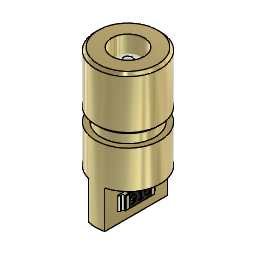
5mW (Autodesk Fusion 360 design; units mm, degrees)
Autodesk Fusion 360 part; units mm, degrees
note: some values were not read from the file. Set by a fixed rule: which sketch regions a step uses.
sketch "Sketch1" plane through (0, 0, 0) normal (0, 0, 1) x (1, 0, 0)
  circle A0 centre (0, 0) radius 3
  dimension "d1" = 6
  constraint coincident A0.centre origin
  measures "d1" diameter of A0
extrude "Extrude1" add sketch "Sketch1" along normal blind 7 makes body 1
sketch "Sketch2" plane through (0, 0, 7) normal (0, 0, 1) x (-1, 0, 0)
  circle A0 centre (0, 0) radius 3
  circle A1 centre (0, 0) radius 2.5
  dimension "d4" = 5
  constraint concentric A0 A1
  measures "d4" diameter of A1
extrude "Extrude2" add sketch "Sketch2" along normal blind 1 contours A1 bodies 1
sketch "Sketch3" plane through (0, 0, 8) normal (0, 0, 1) x (-1, 0, 0)
  circle A0 centre (0, 0) radius 2.5
  circle A1 centre (0, 0) radius 3
  dimension "d7" = 6
  constraint concentric A0 A1
  measures "d7" diameter of A1
extrude "Extrude3" add sketch "Sketch3" along normal blind 5 contours A0 | A1 bodies 1
sketch "Sketch4" plane through (0, 0, 0) normal (0, 0, -1) x (1, 0, 0)
  circle A0 centre (0, 0) radius 3
  line L0 (-0.75, 2.9047) -> (-0.75, -2.9047)
  line L1 (0.75, 2.9047) -> (0.75, -2.9047)
  dimension "d10" = 0.75
  dimension "d11" = 0.75
  constraint coincident A0 L0.start
  constraint coincident A0 L0.end
  constraint vertical L0
  constraint coincident A0 L1.start
  constraint coincident A0 L1.end
  constraint parallel L0 L1
  measures "d10" distance of A0.centre L0
  measures "d11" distance of A0.centre L1
extrude "Extrude4" cut sketch "Sketch4" against normal blind 3.5 contours A0 L1 | A0 L0 bodies 1
sketch "Sketch5" plane through (0, 0, 13) normal (0, 0, 1) x (-1, 0, 0)
  circle A0 centre (0, 0) radius 3
  circle A1 centre (0, 0) radius 1.5
  dimension "d14" = 3
  constraint coincident A0.centre A1.centre
  measures "d14" diameter of A1
extrude "Extrude5" cut sketch "Sketch5" against normal blind 3 contours A1 bodies 1
sketch "Sketch6" plane through (0, 0, 10) normal (0, 0, 1) x (-1, 0, 0)
  circle A0 centre (0, 0) radius 1.5
  circle A1 centre (0, 0) radius 1.4
  dimension "d17" = 2.8
  constraint concentric A0 A1
  measures "d17" diameter of A1
extrude "Extrude6" add sketch "Sketch6" along normal blind 2 separate body contours A1 makes body 2
fillet "Fillet1" radius 1 1 edges at (1.3053, 0.5063, 12) on bodies 2
chamfer "Chamfer1" distance 0.25 angle 45 2 edges at (2.797, 1.0848, 13) (2.797, 1.0848, 8) on bodies 1
sketch "Sketch7" plane through (-0.75, 0, 0) normal (-1, 0, 0) x (0, -1, 0)
  line L0 (-2.9047, 0) -> (2.9047, 0)
  line L1 (2.9047, 0) -> (2.9047, 3.5)
  line L2 (2.9047, 3.5) -> (-2.9047, 3.5)
  line L3 (-2.9047, 3.5) -> (-2.9047, 0)
  circle A0 centre (0, 1.6) radius 1
  dimension "d23" = 2
  dimension "d48" = 2.9047
  dimension "d49" = 1.6
  measures "d23" diameter of A0
  measures "d48" distance of L1 A0.centre
  measures "d49" distance of L0 A0.centre
extrude "Extrude7" add sketch "Sketch7" along normal blind 0.5 contours A0 bodies 1
fillet "Fillet2" radius 0.75 1 edges at (-1.25, 0.9323, 1.2384) on bodies 1
sketch "Sketch8" plane through (0.75, 0, 0) normal (1, 0, 0) x (0, 1, 0)
  line L0 (-2.9047, 0) -> (2.9047, 0)
  line L1 (2.9047, 0) -> (2.9047, 3.5)
  line L2 (2.9047, 3.5) -> (-2.9047, 3.5)
  line L3 (-2.9047, 3.5) -> (-2.9047, 0)
  line L4 (1.75, 1.0641) -> (-1.75, 1.0641)
  line L5 (-1.75, 1.0641) -> (-1.75, 2.3141)
  line L6 (-1.75, 2.3141) -> (1.75, 2.3141)
  line L7 (1.75, 2.3141) -> (1.75, 1.0641)
  line L8 (1.75, 1.0641) -> (-1.75, 2.3141) construction
  line L9 (-1.75, 1.0641) -> (1.75, 2.3141) construction
  line L10 (-1.75, 2.3141) -> (-1.375, 2.3141)
  line L11 (-1.375, 2.3141) -> (-1.375, 1.0641)
  line L12 (-1.375, 1.0641) -> (-1.75, 1.0641)
  line L13 (-1.75, 1.0641) -> (-1.75, 2.3141)
  line L14 (1.75, 2.3141) -> (1.375, 2.3141)
  line L15 (1.375, 2.3141) -> (1.375, 1.0641)
  line L16 (1.375, 1.0641) -> (1.75, 1.0641)
  line L17 (1.75, 1.0641) -> (1.75, 2.3141)
  line L18 (-1.375, 2.3141) -> (-1, 2.3141)
  line L19 (-1, 2.3141) -> (-1, 1.0641)
  line L20 (-1, 1.0641) -> (-1.375, 1.0641)
  line L21 (-1.375, 1.0641) -> (-1.375, 2.3141)
  line L22 (1.375, 2.3141) -> (1, 2.3141)
  line L23 (1, 2.3141) -> (1, 1.0641)
  line L24 (1, 1.0641) -> (1.375, 1.0641)
  line L25 (1.375, 1.0641) -> (1.375, 2.3141)
  line L26 (-1, 2.3141) -> (1, 2.3141)
  line L27 (1, 2.3141) -> (1, 2.3151)
  line L28 (1, 2.3151) -> (-1, 2.3151)
  line L29 (-1, 2.3151) -> (-1, 2.3141)
  line L30 (1, 1.0641) -> (-1, 1.0641)
  line L31 (-1, 1.0641) -> (-1, 1.0631)
  line L32 (-1, 1.0631) -> (1, 1.0631)
  line L33 (1, 1.0631) -> (1, 1.0641)
  line L34 (-1, 2.3141) -> (1, 2.3141)
  line L35 (1, 2.3141) -> (1, 2.314)
  line L36 (1, 2.314) -> (-1, 2.314)
  line L37 (-1, 2.314) -> (-1, 2.3141)
  line L38 (-1, 1.0641) -> (1, 1.0641)
  line L39 (1, 1.0641) -> (1, 1.0642)
  line L40 (1, 1.0642) -> (-1, 1.0642)
  line L41 (-1, 1.0642) -> (-1, 1.0641)
  point P0 (0, 1.6891)
  dimension "d28" = 3.5
  dimension "d29" = 1.25
  dimension "d30" = 0.375
  dimension "d31" = 1.25
  dimension "d32" = 0.375
  dimension "d33" = 0.375
  dimension "d34" = 0.375
  dimension "d50" = 2.9047
  dimension "d51" = 1.6891
  dimension "d52" = 0.001
  dimension "d53" = 2
  dimension "d54" = 0.001
  dimension "d55" = 0.0001
  dimension "d56" = 0.0001
  constraint horizontal L4
  constraint perpendicular L4 L5
  constraint parallel L4 L6
  constraint parallel L5 L7
  constraint coincident L8 P0
  constraint coincident L9 P0
  constraint horizontal L10
  constraint vertical L11
  constraint horizontal L12
  constraint vertical L13
  constraint horizontal L14
  constraint vertical L15
  constraint horizontal L16
  constraint vertical L17
  constraint coincident L4 L15.end
  constraint horizontal L18
  constraint vertical L19
  constraint horizontal L20
  constraint vertical L21
  constraint coincident L4 L19.end
  constraint horizontal L22
  constraint vertical L23
  constraint horizontal L24
  constraint vertical L25
  constraint coincident L4 L23.end
  constraint horizontal L26
  constraint vertical L27
  constraint horizontal L28
  constraint vertical L29
  constraint coincident L23 L27.end
  constraint horizontal L30
  constraint vertical L31
  constraint horizontal L32
  constraint vertical L33
  constraint horizontal L34
  constraint vertical L35
  constraint horizontal L36
  constraint vertical L37
  constraint coincident L23 L35.end
  constraint horizontal L38
  constraint vertical L39
  constraint horizontal L40
  constraint vertical L41
  constraint coincident L23 L39.end
  measures "d28" distance of L5.end L6.end
  measures "d29" distance of L4.end L5.end
  measures "d30" distance of L5.end L10.end
  measures "d31" distance of L5.end L4.end
  measures "d32" distance of L6.end L14.end
  measures "d33" distance of L10.end L18.end
  measures "d34" distance of L14.end L22.end
  measures "d50" distance of L1 P0
  measures "d51" distance of L0 P0
  measures "d52" distance of L18.end L28.end
  measures "d53" distance of L23.end L19.end
  measures "d54" distance of L23.end L32.end
  measures "d55" distance of L18.end L36.end
  measures "d56" distance of L19.end L40.end
extrude "Extrude8" add sketch "Sketch8" along normal blind 0.15 contours L4 L6 L7 L14 L15 L16 L17 L25 | L4 L5 L6 L10 L11 L12 L13 L21 bodies 1
extrude "Extrude9" add sketch "Sketch8" along normal blind 0.4 contours L4 L6 L15 L22 L23 L24 L25 | L4 L6 L11 L18 L19 L20 L21 bodies 1
extrude "Extrude10" add sketch "Sketch8" along normal blind 0.4001 contours L4 L6 L19 L23 L26 L28 L30 L32 L34 L36 L38 L40 bodies 1
fillet "Fillet3" radius 0.15 4 edges at (0.9, -1.75, 1.6891) (0.9, 1.75, 1.6891) (0.9, -1.375, 1.6891) (0.9, 1.375, 1.6891) on bodies 1
fillet "Fillet3" radius 0.05 8 edges at (1.15, 1.375, 1.6891) (1.15, 1.1875, 1.0641) (1.15, -1.1875, 1.0641) (1.15, -1.375, 1.6891) (1.15, -1.1875, 2.3141) (1.15, 1.1875, 2.3141) (1.1501, 0, 1.0631) (1.1501, 0, 2.3151) on bodies 1
sketch "Sketch9" plane through (1.1501, 0, 0) normal (1, 0, 0) x (0, 1, 0)
  line L0 (1, 1.1131) -> (1, 2.2651)
  line L1 (-0.5459, 1.3459) -> (0.5541, 1.3459) construction
  line L2 (0.5541, 1.3459) -> (0.5541, 2.0459) construction
  line L3 (0.5541, 2.0459) -> (-0.5459, 2.0459) construction
  line L4 (-0.5459, 2.0459) -> (-0.5459, 1.3459) construction
  line L5 (1, 2.2651) -> (-1, 2.2651)
  line L6 (-1, 1.1131) -> (1, 1.1131)
  line L7 (-1, 2.2651) -> (-1, 1.1131)
  line L8 (1, 2.2651) -> (-1, 2.2651)
  line L9 (-1, 2.2651) -> (-1, 1.1131)
  line L10 (-1, 1.1131) -> (1, 1.1131)
  line L11 (1, 1.1131) -> (1, 2.2651)
  dimension "d45" = 0.75
  text T0 "910" font "Verdana" height 0.75 align centre middle in box 1.1 x 0.7 at (-0.5459, 1.3459) x (1, 0) y (0, 1) spacing 1
extrude "Extrude11" add sketch "Sketch9" along normal blind 0.001 text T0 bodies 1
combine "Combine2" operation add target body 1 tool bodies 2
equation "d29 = d31"
equation "d32 = d30"
equation "d33 = d30"
equation "d34 = d33"
named bodies: "5mW"
